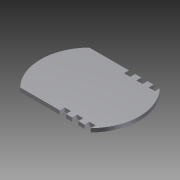
# Autodesk Inventor part: base
Saved by Autodesk Inventor 2012 (Build 160160000, 160)
## iProperties
Created: 2013-01-02
Part Number: base
Material: Default
Document SubType Name: Modeling
Designer: asimov
Density: 1 g/cm^3
Author: asimov
Autodesk Inventor part; units mm, degrees
ref_plane "YZ Plane" through (0, 0, 0) normal (1, 0, 0) x (0, 1, 0)
ref_plane "XZ Plane" through (0, 0, 0) normal (0, 1, 0) x (-1, 0, 0)
ref_plane "XY Plane" through (0, 0, 0) normal (0, 0, 1) x (1, 0, 0)
sketch "Sketch1" plane through (0, 0, 0) normal (0, 0, 1) x (1, 0, 0)
  line L0 (0, 28) -> (-28.5657, 28)
  line L1 (-42.7333, 0) -> (57.4636, 0) construction
  line L2 (0, -28) -> (-28.5657, -28)
  arc A0 (-28.5657, 28) -> (-28.5657, -28) centre (0, 0) ccw
  arc A1 (28.5657, -28) -> (28.5657, 28) centre (0, 0) ccw
  line L3 (28.5657, 28) -> (28.5657, 24)
  line L4 (28.5657, 24) -> (23.5657, 24)
  line L5 (23.5657, 24) -> (23.5657, 28)
  line L6 (23.5657, 28) -> (18.5657, 28)
  line L7 (18.5657, 28) -> (18.5657, 24)
  line L8 (18.5657, 24) -> (13.5657, 24)
  line L9 (13.5657, 24) -> (13.5657, 28)
  line L10 (13.5657, 28) -> (8.5657, 28)
  line L11 (8.5657, 28) -> (8.5657, 24)
  line L12 (8.5657, 24) -> (3.5657, 24)
  line L13 (3.5657, 24) -> (3.5657, 28)
  line L14 (0, 28) -> (3.5657, 28)
  line L15 (8.5657, 28) -> (13.5657, 28)
  line L16 (28.5657, -28) -> (28.5657, -24)
  line L17 (28.5657, -24) -> (23.5657, -24)
  line L18 (23.5657, -24) -> (23.5657, -28)
  line L19 (23.5657, -28) -> (18.5657, -28)
  line L20 (18.5657, -28) -> (18.5657, -24)
  line L21 (18.5657, -24) -> (13.5657, -24)
  line L22 (13.5657, -24) -> (13.5657, -28)
  line L23 (13.5657, -28) -> (8.5657, -28)
  line L24 (8.5657, -28) -> (8.5657, -24)
  line L25 (8.5657, -24) -> (3.5657, -24)
  line L26 (3.5657, -24) -> (3.5657, -28)
  line L27 (8.5657, -28) -> (13.5657, -28)
  line L28 (0, -28) -> (3.5657, -28)
  line L29 (8.5657, -28) -> (13.5657, -28)
  line L30 (18.5657, -28) -> (23.5657, -28)
  dimension "d2" = 40
  dimension "d3" = 40
  dimension "d4" = 4
  dimension "d9" = 5
  dimension "d17" = 4
  dimension "d18" = 4
  dimension "d20" = 4
  dimension "d21" = 4
  constraints: 62 end point, 15 perpendicular, 14 symmetric about line, 4 parallel, 4 point on circle, 2 centre point, 2 collinear, 1 coincident
  measures "d2" radius of A1
  measures "d3" radius of A0
  measures "d4" distance of L3.start L3.end
  measures "d9" distance of L3.end L4.end
  measures "d17" distance of L12.end L13.end
  measures "d18" distance of L4.end L5.end
  measures "d20" distance of L10.end L11.end
  measures "d21" distance of L8.end L9.end
extrude "Extrusion1" add sketch "Sketch1" along normal blind 3
equation "\"d3\" = d2"
equation "\"d17\" = d4"
equation "\"d18\" = d4"
equation "\"d20\" = d4"
equation "\"d21\" = d4"
body "Solid1"
